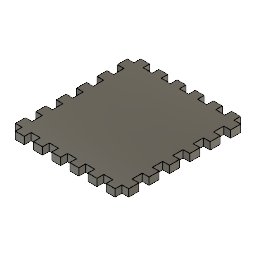
RetroconsoleBottom (Autodesk Fusion 360 design; units mm, degrees)
Autodesk Fusion 360 part; units mm, degrees
sketch "Sketch1" plane through (0, 0, 0) normal (0, 0, 1) x (1, 0, 0)
  line L0 (0, 0) -> (74, 0)
  line L1 (74, 0) -> (74, 83)
  line L2 (74, 83) -> (0, 83)
  line L3 (0, 83) -> (0, 0)
  dimension "d6" = 74
  dimension "d7" = 83
  constraint horizontal L0
  constraint vertical L1
  constraint horizontal L2
  constraint vertical L3
  constraint coincident L0.start L3.end
  measures "d6" distance of L0.start L0.end
  measures "d7" distance of L0.start L2.end
extrude "Extrude1" add sketch "Sketch1" along normal blind 5
sketch "Sketch2" plane through (0, 0, 0) normal (0, -1, 0) x (1, 0, 0)
  line L0 (0, 0) -> (74, 0)
  line L1 (74, 0) -> (74, 5)
  line L2 (74, 5) -> (0, 5)
  line L3 (0, 5) -> (0, 0)
  line L4 (0, 5) -> (6.7273, 5)
  line L5 (6.7273, 5) -> (6.7273, 0)
  line L6 (6.7273, 0) -> (0, 0)
  line L7 (0, 0) -> (0, 5)
  line L8 (20.1818, 0) -> (13.4545, 0)
  line L9 (13.4545, 0) -> (13.4545, 5)
  line L10 (20.1818, 5) -> (20.1818, 0)
  line L11 (13.4545, 5) -> (20.1818, 5)
  line L12 (33.6364, 0) -> (26.9091, 0)
  line L13 (26.9091, 0) -> (26.9091, 5)
  line L14 (33.6364, 5) -> (33.6364, 0)
  line L15 (26.9091, 5) -> (33.6364, 5)
  line L16 (47.0909, 0) -> (40.3636, 0)
  line L17 (40.3636, 0) -> (40.3636, 5)
  line L18 (47.0909, 5) -> (47.0909, 0)
  line L19 (40.3636, 5) -> (47.0909, 5)
  line L20 (60.5455, 0) -> (53.8182, 0)
  line L21 (53.8182, 0) -> (53.8182, 5)
  line L22 (60.5455, 5) -> (60.5455, 0)
  line L23 (53.8182, 5) -> (60.5455, 5)
  line L24 (74, 0) -> (67.2727, 0)
  line L25 (67.2727, 0) -> (67.2727, 5)
  line L26 (74, 5) -> (74, 0)
  line L27 (67.2727, 5) -> (74, 5)
  dimension "d10" = 6.7273
  dimension "d13" = 67.2727
  dimension "d14" = 0
  constraint horizontal L4
  constraint vertical L5
  constraint horizontal L6
  constraint vertical L7
  constraint coincident L0 L5.end
  constraint coincident L2.end L3.start
  measures "d10" distance of L2.end L4.end
extrude "Extrude2" add sketch "Sketch2" along normal blind 5 contours L0 L2 L3 L4 L5 L6 L7 | L0 L2 L8 L9 L10 L11 | L0 L2 L12 L13 L14 L15 | L0 L2 L16 L17 L18 L19 | L0 L2 L20 L21 L22 L23 | L0 L1 L2 L24 L25 L26 L27
sketch "Sketch3" plane through (0, 83, 0) normal (0, 1, 0) x (-1, 0, 0)
  line L0 (-74, 0) -> (0, 0)
  line L1 (0, 0) -> (0, 5)
  line L2 (0, 5) -> (-74, 5)
  line L3 (-74, 5) -> (-74, 0)
  line L4 (-74, 5) -> (-67.2727, 5)
  line L5 (-67.2727, 5) -> (-67.2727, 0)
  line L6 (-67.2727, 0) -> (-74, 0)
  line L7 (-74, 0) -> (-74, 5)
  line L8 (-53.8182, 0) -> (-60.5455, 0)
  line L9 (-60.5455, 0) -> (-60.5455, 5)
  line L10 (-53.8182, 5) -> (-53.8182, 0)
  line L11 (-60.5455, 5) -> (-53.8182, 5)
  line L12 (-40.3636, 0) -> (-47.0909, 0)
  line L13 (-47.0909, 0) -> (-47.0909, 5)
  line L14 (-40.3636, 5) -> (-40.3636, 0)
  line L15 (-47.0909, 5) -> (-40.3636, 5)
  line L16 (-26.9091, 0) -> (-33.6364, 0)
  line L17 (-33.6364, 0) -> (-33.6364, 5)
  line L18 (-26.9091, 5) -> (-26.9091, 0)
  line L19 (-33.6364, 5) -> (-26.9091, 5)
  line L20 (-13.4545, 0) -> (-20.1818, 0)
  line L21 (-20.1818, 0) -> (-20.1818, 5)
  line L22 (-13.4545, 5) -> (-13.4545, 0)
  line L23 (-20.1818, 5) -> (-13.4545, 5)
  line L24 (0, 0) -> (-6.7273, 0)
  line L25 (-6.7273, 0) -> (-6.7273, 5)
  line L26 (0, 5) -> (0, 0)
  line L27 (-6.7273, 5) -> (0, 5)
  dimension "d17" = 6.7273
  dimension "d20" = 67.2727
  dimension "d21" = 0
  constraint horizontal L4
  constraint vertical L5
  constraint horizontal L6
  constraint vertical L7
  constraint coincident L0 L5.end
  constraint coincident L2.end L3.start
  measures "d17" distance of L2.end L4.end
extrude "Extrude3" add sketch "Sketch3" along normal blind 5 contours L0 L2 L3 L4 L5 L6 L7 | L0 L2 L8 L9 L10 L11 | L0 L2 L12 L13 L14 L15 | L0 L2 L16 L17 L18 L19 | L0 L2 L20 L21 L22 L23 | L0 L1 L2 L24 L25 L26 L27
sketch "Sketch4" plane through (0, 0, 0) normal (1, 0, 0) x (0, 1, 0)
  line L0 (0, 0) -> (7.5455, 0)
  line L1 (7.5455, 0) -> (7.5455, 5)
  line L2 (7.5455, 5) -> (0, 5)
  line L3 (0, 5) -> (0, 0)
  line L4 (88, 5) -> (-5, 5)
  line L5 (15.0909, 0) -> (22.6364, 0)
  line L6 (22.6364, 0) -> (22.6364, 5)
  line L7 (22.6364, 5) -> (15.0909, 5)
  line L8 (15.0909, 5) -> (15.0909, 0)
  line L9 (30.1818, 0) -> (37.7273, 0)
  line L10 (37.7273, 0) -> (37.7273, 5)
  line L11 (37.7273, 5) -> (30.1818, 5)
  line L12 (30.1818, 5) -> (30.1818, 0)
  line L13 (45.2727, 0) -> (52.8182, 0)
  line L14 (52.8182, 0) -> (52.8182, 5)
  line L15 (52.8182, 5) -> (45.2727, 5)
  line L16 (45.2727, 5) -> (45.2727, 0)
  line L17 (60.3636, 0) -> (67.9091, 0)
  line L18 (67.9091, 0) -> (67.9091, 5)
  line L19 (67.9091, 5) -> (60.3636, 5)
  line L20 (60.3636, 5) -> (60.3636, 0)
  line L21 (75.4545, 0) -> (83, 0)
  line L22 (83, 0) -> (83, 5)
  line L23 (83, 5) -> (75.4545, 5)
  line L24 (75.4545, 5) -> (75.4545, 0)
  dimension "d24" = 7.5455
  dimension "d27" = 75.4545
  dimension "d28" = 0
  constraint horizontal L0
  constraint vertical L1
  constraint horizontal L2
  constraint vertical L3
  constraint coincident L1.end L4
  constraint coincident L0.start L3.end
  measures "d24" distance of L1.end L2.end
extrude "Extrude4" add sketch "Sketch4" against normal blind 5
sketch "Sketch5" plane through (74, 0, 0) normal (1, 0, 0) x (0, 1, 0)
  line L0 (-5, 0) -> (88, 0)
  line L1 (88, 0) -> (88, 5)
  line L2 (88, 5) -> (-5, 5)
  line L3 (-5, 5) -> (-5, 0)
  line L4 (0, 0) -> (7.5455, 0)
  line L5 (7.5455, 0) -> (7.5455, 5)
  line L6 (7.5455, 5) -> (0, 5)
  line L7 (0, 5) -> (0, 0)
  line L8 (15.0909, 0) -> (22.6364, 0)
  line L9 (22.6364, 0) -> (22.6364, 5)
  line L10 (22.6364, 5) -> (15.0909, 5)
  line L11 (15.0909, 5) -> (15.0909, 0)
  line L12 (30.1818, 0) -> (37.7273, 0)
  line L13 (37.7273, 0) -> (37.7273, 5)
  line L14 (37.7273, 5) -> (30.1818, 5)
  line L15 (30.1818, 5) -> (30.1818, 0)
  line L16 (45.2727, 0) -> (52.8182, 0)
  line L17 (52.8182, 0) -> (52.8182, 5)
  line L18 (52.8182, 5) -> (45.2727, 5)
  line L19 (45.2727, 5) -> (45.2727, 0)
  line L20 (60.3636, 0) -> (67.9091, 0)
  line L21 (67.9091, 0) -> (67.9091, 5)
  line L22 (67.9091, 5) -> (60.3636, 5)
  line L23 (60.3636, 5) -> (60.3636, 0)
  line L24 (75.4545, 0) -> (83, 0)
  line L25 (83, 0) -> (83, 5)
  line L26 (83, 5) -> (75.4545, 5)
  line L27 (75.4545, 5) -> (75.4545, 0)
  dimension "d31" = 7.5455
  dimension "d34" = 75.4545
  dimension "d35" = 0
  constraint horizontal L4
  constraint vertical L5
  constraint horizontal L6
  constraint vertical L7
  constraint coincident L2 L5.end
  constraint coincident L4.start L7.end
  measures "d31" distance of L5.end L6.end
extrude "Extrude5" add sketch "Sketch5" along normal blind 5 contours L0 L2 L4 L5 L6 L7 | L0 L2 L8 L9 L10 L11 | L0 L2 L12 L13 L14 L15 | L0 L2 L16 L17 L18 L19 | L0 L2 L20 L21 L22 L23 | L0 L2 L24 L25 L26 L27
extrude "Extrude6" add 1 faces at (38.1212, 25.1515, 5) along direction (0, 0, 1) blind 0.5
sketch "Sketch6" plane through (79, 0, 0) normal (1, 0, 0) x (0, 1, 0)
  line L0 (75.4545, 5.5) -> (75.4545, 0)
  line L1 (75.4545, 0) -> (83, 0)
  line L2 (83, 0) -> (83, 5.5)
  line L3 (83, 5.5) -> (75.4545, 5.5)
sketch "Sketch7" plane through (0, 0, 0) normal (0, 0, 1) x (1, 0, 0)
  line L0 (79, 75.4545) -> (79, 83) construction
  line L1 (79, 83) -> (91, 83) construction
  line L2 (91, 83) -> (101, 83)
  line L3 (101, 83) -> (101, -6)
  line L4 (101, -6) -> (91, -6)
  line L5 (91, -6) -> (91, 83)
  line L6 (91, 83) -> (101, 83)
  line L7 (101, 83) -> (101, 89)
  line L8 (101, 89) -> (91, 89)
  line L9 (91, 89) -> (91, 83)
  line L10 (91, 83) -> (85, 83)
  line L11 (85, 83) -> (85, 89)
  line L12 (85, 89) -> (91, 89)
  line L13 (91, 89) -> (91, 83)
  line L14 (91, -6) -> (85, -6)
  line L15 (85, -6) -> (85, 0)
  line L16 (85, 0) -> (91, 0)
  line L17 (91, 0) -> (91, -6)
  point P0 (79, 83)
  dimension "d40" = 12
  dimension "d41" = 89
  dimension "d42" = 10
  dimension "d43" = 6
  dimension "d44" = 6
  dimension "d45" = 6
  dimension "d46" = 6
  dimension "d47" = 6
  constraint coincident P0 L0.end
  constraint perpendicular L0 L1
  constraint horizontal L2
  constraint vertical L3
  constraint horizontal L4
  constraint vertical L5
  constraint horizontal L6
  constraint vertical L7
  constraint horizontal L8
  constraint vertical L9
  constraint horizontal L10
  constraint vertical L11
  constraint horizontal L12
  constraint vertical L13
  constraint horizontal L14
  constraint vertical L15
  constraint horizontal L16
  constraint vertical L17
  measures "d40" distance of P0 L1.end
  measures "d41" distance of L1.end L4.end
  measures "d42" distance of L1.end L2.end
  measures "d43" distance of L1.end L8.end
  measures "d44" distance of L1.end L10.end
  measures "d45" distance of L1.end L8.end
  measures "d46" distance of L4.end L14.end
  measures "d47" distance of L4.end L16.end
sketch "Sketch8" plane through (91, 0, 0) normal (-1, 0, 0) x (0, -1, 0)
  line L0 (-82, 0) -> (0, 0)
  line L1 (0, 0) -> (0, 6.5)
  line L2 (0, 6.5) -> (-82, 6.5)
  line L3 (-82, 6.5) -> (-82, 0)
  line L4 (-74.4545, 6.5) -> (-66.9091, 6.5)
  line L5 (-66.9091, 6.5) -> (-66.9091, 0)
  line L6 (-66.9091, 0) -> (-74.4545, 0)
  line L7 (-74.4545, 0) -> (-74.4545, 6.5)
  line L8 (-51.8182, 0) -> (-59.3636, 0)
  line L9 (-59.3636, 0) -> (-59.3636, 6.5)
  line L10 (-51.8182, 6.5) -> (-51.8182, 0)
  line L11 (-59.3636, 6.5) -> (-51.8182, 6.5)
  line L12 (-36.7273, 0) -> (-44.2727, 0)
  line L13 (-44.2727, 0) -> (-44.2727, 6.5)
  line L14 (-36.7273, 6.5) -> (-36.7273, 0)
  line L15 (-44.2727, 6.5) -> (-36.7273, 6.5)
  line L16 (-21.6364, 0) -> (-29.1818, 0)
  line L17 (-29.1818, 0) -> (-29.1818, 6.5)
  line L18 (-21.6364, 6.5) -> (-21.6364, 0)
  line L19 (-29.1818, 6.5) -> (-21.6364, 6.5)
  line L20 (-6.5455, 0) -> (-14.0909, 0)
  line L21 (-14.0909, 0) -> (-14.0909, 6.5)
  line L22 (-6.5455, 6.5) -> (-6.5455, 0)
  line L23 (-14.0909, 6.5) -> (-6.5455, 6.5)
  dimension "d50" = 7.5455
  dimension "d51" = 7.5455
  dimension "d54" = 60.3636
  dimension "d55" = 0
  constraint horizontal L4
  constraint vertical L5
  constraint horizontal L6
  constraint vertical L7
  constraint coincident L0 L5.end
  constraint coincident L2 L4.start
  measures "d50" distance of L2.end L4.start
  measures "d51" distance of L4.start L4.end
sketch "Sketch9" plane through (0, 0, 0) normal (0, 0, 1) x (1, 0, 0)
equation "paksus = 5 mm"
equation "laius = 74 mm"
equation "pikkus = 83 mm"
equation "laius_tapp = laius / 11"
equation "pikkus_tapp = pikkus / 11"
equation "d6 = laius"
equation "d7 = pikkus"
equation "d8 = paksus"
equation "d10 = laius_tapp"
equation "d13 = laius - laius_tapp"
equation "d15 = paksus"
equation "d17 = laius_tapp"
equation "d20 = laius - laius_tapp"
equation "d22 = paksus"
equation "d24 = pikkus_tapp"
equation "d27 = pikkus - pikkus_tapp"
equation "d29 = -paksus"
equation "d31 = pikkus_tapp"
equation "d34 = pikkus - pikkus_tapp"
equation "d36 = paksus"
equation "d41 = pikkus + 6 mm"
equation "d50 = pikkus_tapp"
equation "d51 = pikkus_tapp"
equation "d54 = pikkus - pikkus_tapp * 3"
